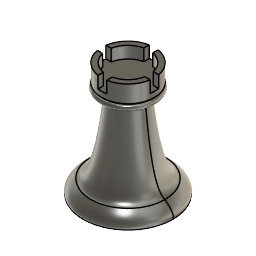
Tura (Autodesk Fusion 360 design; units mm, degrees)
part number: 2026-03-27-15-39-02-789
Autodesk Fusion 360 part; units mm, degrees
sketch "Tura" plane through (0, 0, 0) normal (0, 1, 0) x (1, 0, 0)
  line L0 (0, 0) -> (17, 0)
  line L1 (0, 0) -> (0, -38.5138)
  line L2 (0, -38.5138) -> (0, -35)
  line L3 (0, -38.5138) -> (0, -35)
  line L4 (0, 0) -> (0, -5)
  line L5 (14, -5) -> (0, -5)
  spline S0 degree 5 poles (6.5259, -34) (6.6855, -32.318) (7.0209, -29.0147) (7.5725, -24.2418) (8.412, -18.2671) (9.7194, -11.7648) (11.1016, -7.8229) (12.4226, -5.9311) (13.4497, -5.2188) (14, -5) knots 0 0 0 0 0 0 0.2 0.4 0.6 0.8 1 1 1 1 1 1
  line L6 (12.8092, -5.4735) -> (15.1908, -4.5265)
  spline S1 degree 5 poles (14, -5) (14.3724, -4.7164) (15.065, -4.1591) (15.9469, -3.3525) (16.8041, -2.3367) (17.2264, -1.3701) (17.2496, -0.692) (17.1232, -0.2556) (17.015, -0.0297) (17, 0) knots 0 0 0 0 0 0 0.1 0.2 0.3 0.4 0.415205 0.415205 0.415205 0.415205 0.415205 0.415205
  line L7 (17.1967, -0.3896) -> (16.8033, 0.3896)
  line L8 (0, -37.3622) -> (0, -38.5138)
  line L9 (0, -36) -> (9, -36)
  line L10 (0, -38) -> (0, -36)
  line L11 (8, -40) -> (8, -43)
  line L12 (8, -43) -> (10, -43)
  line L13 (10, -43) -> (10, -36.5)
  line L14 (9.5, -36) -> (9, -36)
  line L15 (0, -36) -> (9.5003, -36)
  line L16 (9.5, -34) -> (0, -34)
  line L17 (0, -34) -> (0, -36)
  arc A0 (9.5005, -34) -> (9.5, -34) centre (9.5, -36.5) ccw
  arc A1 (9.5003, -36) -> (9.5005, -34) centre (9.5003, -35) ccw
  arc A2 (10, -36.5) -> (9.5, -36) centre (9.5, -36.5) ccw
  line L18 (-1.7845, -43) -> (1.4873, -43)
  line L19 (1.4873, -43) -> (1.4873, -38.5138)
  line L20 (1.4873, -38.5138) -> (-1.7845, -38.5138)
  line L21 (-1.7845, -38.5138) -> (-1.7845, -43)
  line L22 (1.4873, -38.5138) -> (8, -38.5138)
  line L23 (8, -38.5138) -> (8, -40)
  point P0 (10, -35)
  dimension "d1" = 17
  dimension "d3" = 10
  dimension "d5" = 3
  dimension "d6" = 2.5
  dimension "d7" = 1
  dimension "d8" = 0.5
  constraint coincident L0.start L1.start
  constraint horizontal L0
  constraint perpendicular L0 L1
  constraint coincident L1 L2.end
  constraint coincident L1 L4.end
  constraint perpendicular L4 L5
  constraint midpoint L5.start L6
  constraint midpoint L0.end L7
  constraint vertical L8
  constraint horizontal L9
  constraint vertical L10
  constraint coincident L1 L9.start
  constraint perpendicular L11 L12
  constraint perpendicular L12 L13
  constraint horizontal L15
  constraint horizontal L16
  constraint vertical L17
  constraint tangent L16 A0
  constraint tangent L15 A1
  constraint tangent A0 A1
  constraint tangent L13 A2
  constraint tangent L14 A2
  constraint coincident S0.start L16
  constraint horizontal L18
  constraint vertical L19
  constraint horizontal L20
  constraint vertical L21
  constraint perpendicular L19 L22
  constraint perpendicular L22 L23
  constraint coincident L20 L1.end
  measures "d1" distance of L0.start L0.end
  measures "d3" distance of L2.end P0
  measures "d5" distance of L11.start L11.end
  measures "d6" radius of A0
  measures "d7" radius of A1
  measures "d8" radius of A2
revolve "Revolve2" add sketch "Tura" angle 360 about axis through (0, 0, 0) along (0, 0, 1) contours L0 L1 L4 L5 S1 | L1 L5 S0 L16 | L1 L2 L3 L9 L15 L16 L17 A0 | L9 L14 L15 A0 A1 | L1 L2 L3 L8 L9 L10 L11 L12 L13 L15 A0 L20 L22 L23 | L9 L13 L14 L15 A0 A2
extrude "Extrude2" cut sketch "Tura" along normal blind 10 contours L18 L19 L20 L21
pattern_circular "C-Pattern1" count 4 over 360 about axis through (0, 0, 0) along (0, 0, 1) of "Extrude2"
named bodies: "Tura"
